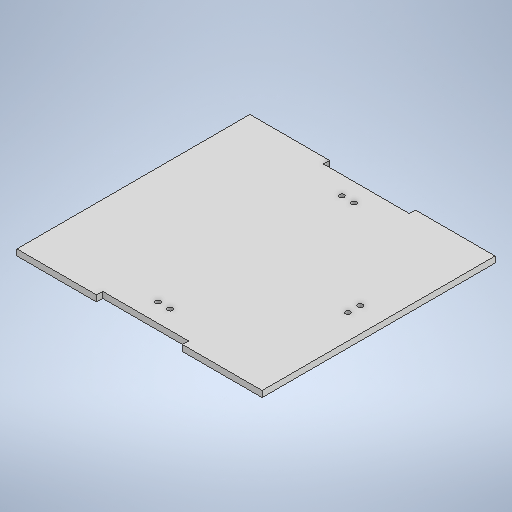
# Autodesk Inventor part: top
Saved by Autodesk Inventor 2025.3 (Build 293356030, 356C)
## iProperties
Created: 2026-06-26
Part Number: top
Material: Generic
Document SubType Name: Modeling
Designer: user
Density: 1 g/cm^3
Appearance: Default
Author: user
Autodesk Inventor part; units mm, degrees
ref_plane "YZ Plane" through (0, 0, 0) normal (1, 0, 0) x (0, 1, 0)
ref_plane "XZ Plane" through (0, 0, 0) normal (0, 1, 0) x (-1, 0, 0)
ref_plane "XY Plane" through (0, 0, 0) normal (0, 0, 1) x (1, 0, 0)
sketch "Sketch1" plane through (0, 0, 0) normal (0, 1, 0) x (-1, 0, 0)
  line L0 (0, 0) -> (-200, 0)
  line L1 (-200, 0) -> (-200, -190)
  line L2 (-200, -190) -> (0, -190)
  line L3 (0, -190) -> (0, 0)
  line L4 (-65, 0) -> (-135, 0)
  line L5 (-135, 0) -> (-135, -5)
  line L6 (-135, -5) -> (-65, -5)
  line L7 (-65, -5) -> (-65, 0)
  line L8 (-200, -95) -> (0, -95) construction
  line L9 (-65, -190) -> (-135, -190)
  line L10 (-135, -190) -> (-135, -185)
  line L11 (-135, -185) -> (-65, -185)
  line L12 (-65, -185) -> (-65, -190)
  line L13 (-200, -215) -> (-200, -15)
  dimension "d0" = 200
  dimension "d2" = 70
  dimension "d3" = 5
  dimension "d11" = 0
  dimension "d13" = 190
  constraints: 28 end point, 4 parallel, 4 symmetric about line, 2 horizontal, 2 midpoint, 2 perpendicular, 1 point on line
  measures "d0" distance of L2.end L1.end
  measures "d2" distance of L6.end L5.end
  measures "d3" distance of L5.end L4.end
  measures "d11" distance between parallel lines of L0 L4
  measures "d13" distance between parallel lines of L0 L2
extrude "Extrusion1" add sketch "Sketch1" along normal blind 5 contours L3 L2 L12 L11 L10 L1 L0 L5 L6 L7
sketch "Sketch2" plane through (0, 5, 0) normal (0, 1, 0) x (1, 0, 0)
  line L0 (0, 0) -> (65, 0) projected
  line L1 (135, 0) -> (200, 0) projected
  line L2 (65, 0) -> (65, 5) projected
  line L3 (0, 190) -> (0, 0) projected
  line L4 (0, 95) -> (200, 95)
  point P0 (95, 20)
  point P1 (105, 20)
  point P2 (95, 170)
  point P3 (105, 170)
  dimension "d22" = 20
  dimension "d23" = 10
  dimension "d24" = 20
  dimension "d25" = 30
  constraints: 2 end point, 2 symmetric about line, 1 horizontal, 1 midpoint
  measures "d22" distance from line of L1 point (105, 20)
  measures "d23" distance of point (105, 20) point (95, 20)
  measures "d24" distance from line of L0 point (95, 20)
  measures "d25" distance from line of L2 point (95, 20)
hole "Hole1" at (95, 5, -20) at (105, 5, -20) at (95, 5, -170) at (105, 5, -170) direction (0, -1, 0) diameter 4 end through all
sketch "Sketch5" plane through (0, 5, 0) normal (0, 1, 0) x (1, 0, 0)
  line L0 (200, 0) -> (200, 190) projected
  line L1 (200, 190) -> (135, 190) projected
  point P0 (0, 0)
  point P1 (180, 90)
  point P2 (180, 100)
  dimension "d51" = 20
  dimension "d52" = 20
  dimension "d53" = 10
  dimension "d54" = 90
  measures "d51" distance from line of point (180, 100) L0
  measures "d52" distance from line of L0 point (180, 90)
  measures "d53" distance of point (180, 90) point (180, 100)
  measures "d54" distance from line of L1 point (180, 100)
hole "Hole4" at (180, 5, -90) at (180, 5, -100) direction (0, -1, 0) diameter 4 end through all
body "Solid1"
